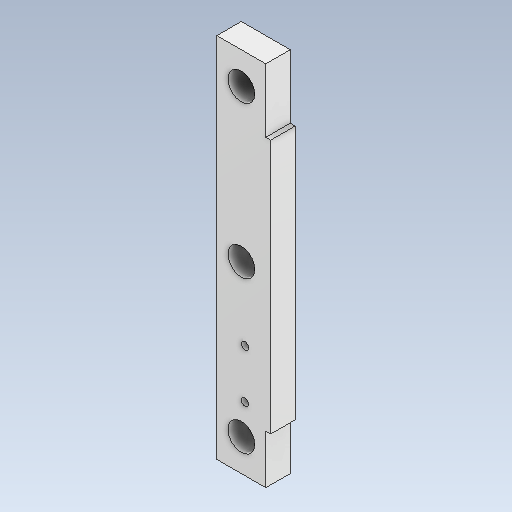
# Autodesk Inventor part: Z_endstop_mount
Saved by Autodesk Inventor 2020 (Build 240168000, 168)
## iProperties
Created: 2022-03-31
Part Number: Z_endstop_mount
Material: Tworzywo sztuczne ABS
Document SubType Name: Modeling
Designer: mikoma
Density: 1.06 g/cm^3
Appearance: Gładki — biały
Mass: 3.85411 g
Surface Area: 26.2069 cm^2
Volume: 3.63595 cm^3
Author: mikoma
Autodesk Inventor part; units mm, degrees
ref_plane "YZ Plane" through (0, 0, 0) normal (1, 0, 0) x (0, 1, 0)
ref_plane "XZ Plane" through (0, 0, 0) normal (0, 1, 0) x (-1, 0, 0)
ref_plane "XY Plane" through (0, 0, 0) normal (0, 0, 1) x (1, 0, 0)
sketch "Szkic1" plane through (0, 0, 0) normal (0, 0, 1) x (1, 0, 0)
  line L0 (-5, -37.5) -> (5, -37.5)
  line L1 (5, -37.5) -> (5, 37.5)
  line L2 (5, 37.5) -> (-5, 37.5)
  line L3 (-5, 37.5) -> (-5, -37.5)
  line L4 (-5, -37.5) -> (5, 37.5) construction
  line L5 (5, -37.5) -> (-5, 37.5) construction
  circle A0 centre (0, 31) radius 2.75
  circle A1 centre (0, -31) radius 2.75
  line L6 (6, -27.5) -> (5, -27.5)
  line L7 (5, -27.5) -> (5, 24.5)
  line L8 (5, 24.5) -> (6, 24.5)
  line L9 (6, 24.5) -> (6, -27.5)
  line L10 (6, -27.5) -> (5, 24.5) construction
  line L11 (5, -27.5) -> (6, 24.5) construction
  circle A2 centre (0.75, -24.5) radius 0.75
  circle A3 centre (0.75, -14.5) radius 0.75
  line L12 (-1.5, -13.201) -> (0.75, -11.9019)
  line L13 (0.75, -11.9019) -> (3, -13.201)
  line L14 (3, -13.201) -> (3, -15.799)
  line L15 (3, -15.799) -> (0.75, -17.0981)
  line L16 (0.75, -17.0981) -> (-1.5, -15.799)
  line L17 (-1.5, -15.799) -> (-1.5, -13.201)
  line L18 (-1.5, -23.201) -> (0.75, -21.9019)
  line L19 (0.75, -21.9019) -> (3, -23.201)
  line L20 (3, -23.201) -> (3, -25.799)
  line L21 (3, -25.799) -> (0.75, -27.0981)
  line L22 (0.75, -27.0981) -> (-1.5, -25.799)
  line L23 (-1.5, -25.799) -> (-1.5, -23.201)
  circle A4 centre (0, 0) radius 2.75
  point P0 (0, 0)
  point P1 (5.5, -1.5)
  point P2 (5, -27.5)
  dimension "d0" = 75
  dimension "d1" = 10
  dimension "d2" = 5.5
  dimension "d3" = 31
  dimension "d4" = 31
  dimension "d5" = 10
  dimension "d6" = 13
  dimension "d7" = 1
  dimension "d10" = 1.5
  dimension "d11" = 1.5
  dimension "d12" = 3
  dimension "d13" = 10
  dimension "d15" = 4.5
  dimension "d16" = 4.5
  dimension "d17" = 3
  dimension "d20" = 5.5
  constraints: 48 end point, 5 centre point, 5 midpoint, 4 parallel, 3 coincident, 3 vertical alignment, 2 horizontal, 2 perpendicular, 2 vertical, 1 equal radius, 1 point on line, 26 other
  measures "d0" distance of L0.end L1.end
  measures "d1" distance of L1.end L2.end
  measures "d2" diameter of A0
  measures "d3" distance of point (0, 0) A0.centre
  measures "d4" distance of point (0, 0) A1.centre
  measures "d5" distance between parallel lines of L6 L0
  measures "d6" distance between parallel lines of L2 L8
  measures "d7" distance of L7.end L8.end
  measures "d10" diameter of A3
  measures "d11" diameter of A2
  measures "d12" distance from line of A2.centre L6
  measures "d13" distance of A3.centre A2.centre
  measures "d15" distance between parallel lines of L14 L17
  measures "d16" distance between parallel lines of L20 L23
  measures "d17" distance between parallel lines of L9 L14
  measures "d20" diameter of A4
extrude "Wyciągnięcie proste1" add sketch "Szkic1" along normal blind 5 contours L3 L2 L1 L0 | L1 L8 L9 L6 | L12 L13 L14 L15 L16 L17 | L18 L19 L20 L21 L22 L23
equation "\"d4\" = d3"
